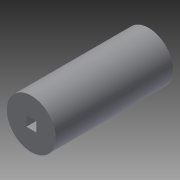
# Autodesk Inventor part: VEX Encoder shaft converter
Saved by Autodesk Inventor 2014 SP1 (Build 180222100, 222)
## iProperties
Created: 2014-02-16
Part Number: VEX Encoder shaft converter
Material: Generic
Document SubType Name: Modeling
Designer: habib asif
Density: 1 g/cm^3
Appearance: Default
Author: habib asif
Autodesk Inventor part; units mm, degrees
ref_plane "YZ Plane" through (0, 0, 0) normal (1, 0, 0) x (0, 1, 0)
ref_plane "XZ Plane" through (0, 0, 0) normal (0, 1, 0) x (-1, 0, 0)
ref_plane "XY Plane" through (0, 0, 0) normal (0, 0, 1) x (1, 0, 0)
sketch "Sketch1" plane through (0, 0, 0) normal (0, 0, 1) x (1, 0, 0)
  circle A0 centre (-0.9432, 0.695) radius 7.9375
  circle A1 centre (-0.9432, 0.695) radius 4.7625
  dimension "d0" = 9.525
  dimension "d1" = 15.875
  constraints: 2 centre point, 1 coincident, 1 other
  measures "d0" diameter of A1
  measures "d1" diameter of A0
extrude "Extrusion1" add sketch "Sketch1" along normal blind 25.4
sketch "Sketch3" plane through (-0.9432, 0.695, 25.4) normal (0, 0, 1) x (1, 0, 0)
  circle A0 centre (0, 0) radius 7.9375 projected
  circle A1 centre (0, 0) radius 7.9375
  constraints: 1 centre point, 1 coincident, 1 concentric
extrude "Extrusion2" add sketch "Sketch3" along normal blind 12.7
sketch "Sketch5" plane through (-0.9432, 0.695, 38.1) normal (0, 0, 1) x (1, 0, 0)
  circle A0 centre (0, 0) radius 7.9375 projected
  line L0 (-1.5875, 1.5875) -> (1.5875, 1.5875)
  line L1 (1.5875, 1.5875) -> (1.5875, -1.5875)
  line L2 (1.5875, -1.5875) -> (-1.5875, -1.5875)
  line L3 (-1.5875, -1.5875) -> (-1.5875, 1.5875)
  point P0 (0, -1.5875)
  point P1 (1.5875, 0)
  dimension "d6" = 3.175
  constraints: 8 end point, 2 midpoint, 2 parallel, 2 perpendicular, 1 horizontal, 1 horizontal alignment, 1 vertical alignment
  measures "d6" distance of L1.end L2.end
extrude "Extrusion3" cut sketch "Sketch5" against normal up to surface (12.7 mm away) contours L0 L1 L2 L3
body "Solid1"
